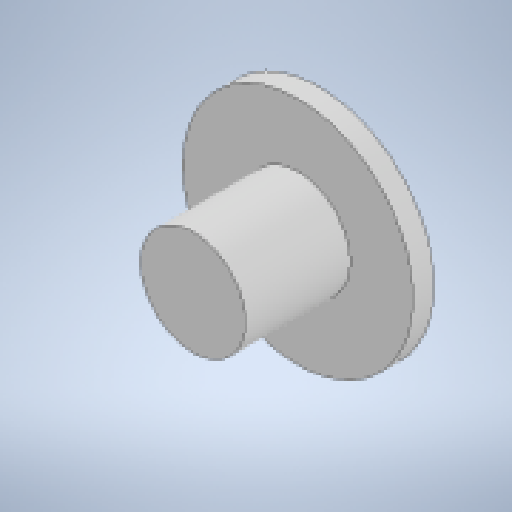
# Autodesk Inventor part: фланец
Saved by Autodesk Inventor 2023.1 (Build 271208000, 208)
## iProperties
Created: 2024-12-17
Part Number: фланец
Material: Типовые
Document SubType Name: Modeling
Designer: DELL
Density: 1 g/cm^3
Appearance: По умолчанию
Author: DELL
Autodesk Inventor part; units mm, degrees
ref_plane "YZ Plane" through (0, 0, 0) normal (1, 0, 0) x (0, 1, 0)
ref_plane "XZ Plane" through (0, 0, 0) normal (0, 1, 0) x (-1, 0, 0)
ref_plane "XY Plane" through (0, 0, 0) normal (0, 0, 1) x (1, 0, 0)
sketch "Эскиз1" plane through (0, 0, 0) normal (0, 0, 1) x (1, 0, 0)
  arc A0 (8.9721, -40.2077) -> (-8.9721, -40.2077) centre (0, -39.5) ccw construction
  line L0 (8.9721, -40.2077) -> (11, -14.5) construction
  arc A1 (11, -14.5) -> (-11, -14.5) centre (0, -14.5) ccw construction
  line L1 (-11, -14.5) -> (-8.9721, -40.2077) construction
  circle A2 centre (0, -14.5) radius 5 construction
  circle A3 centre (0, -14.5) radius 11
  circle A4 centre (0, -14.5) radius 5
  point P0 (0, 0)
  dimension "d0" = 22
  dimension "d1" = 10
  constraints: 2 centre point, 2 coincident
  measures "d0" diameter of A3
  measures "d1" diameter of A4
extrude "Выдавливание1" add sketch "Эскиз1" along normal blind 12 contours A4
sketch "Эскиз2" plane through (0, 0, 0) normal (0, 0, 1) x (1, 0, 0)
  circle A0 centre (0, -14.5) radius 5 projected
  circle A1 centre (0, -14.5) radius 11
  point P0 (0, 0)
  dimension "d4" = 22
  constraints: 1 centre point, 1 coincident
  measures "d4" diameter of A1
extrude "Выдавливание2" add sketch "Эскиз2" along normal blind 2
